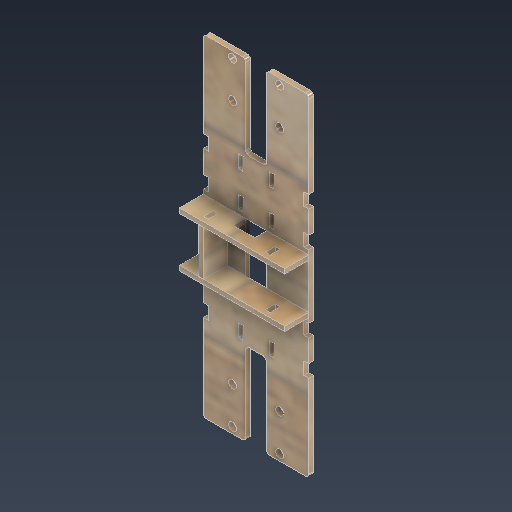
# Autodesk Inventor part: edited
Saved by Autodesk Inventor 2025.3 (Build 293356000, 356)
## iProperties
Created: 2025-09-03
Part Number: edited
Material: 木材 (楓木)
Document SubType Name: Modeling
Designer: 陳泓任
Density: 0.67 g/cm^3
Appearance: 天然楓木 - 深色亮面處理
Author: 陳泓任
Autodesk Inventor part; units mm, degrees
ref_plane "YZ Plane" through (0, 0, 0) normal (1, 0, 0) x (0, 1, 0)
ref_plane "XZ Plane" through (0, 0, 0) normal (0, 1, 0) x (-1, 0, 0)
ref_plane "XY Plane" through (0, 0, 0) normal (0, 0, 1) x (1, 0, 0)
sketch "草圖1" plane through (0, 0, 0) normal (0, 0, 1) x (1, 0, 0)
  line L0 (-33, -104) -> (33, 104) construction
  line L1 (33, -104) -> (-33, 104) construction
  line L2 (0, 128.5379) -> (0, -160.5456) construction
  circle A0 centre (-14.75, 100) radius 2.5
  circle A1 centre (14.75, 100) radius 2.5
  circle A2 centre (14.75, 77) radius 2.5
  circle A3 centre (-14.75, 77) radius 2.5
  line L3 (-33, 49.8787) -> (-30, 49.8787)
  line L4 (-30, 49.8787) -> (-30, 41.8787)
  line L5 (-30, 41.8787) -> (-33, 41.8787)
  line L6 (-33, 102) -> (-33, 49.8787)
  line L7 (-11.2, 49.8787) -> (-8.2, 49.8787)
  line L8 (-8.2, 49.8787) -> (-8.2, 41.8787)
  line L9 (-8.2, 41.8787) -> (-11.2, 41.8787)
  line L10 (-11.2, 41.8787) -> (-11.2, 49.8787)
  line L11 (33, 49.8787) -> (30, 49.8787)
  line L12 (30, 49.8787) -> (30, 41.8787)
  line L13 (30, 41.8787) -> (33, 41.8787)
  line L14 (11.2, 49.8787) -> (8.2, 49.8787)
  line L15 (8.2, 49.8787) -> (8.2, 41.8787)
  line L16 (8.2, 41.8787) -> (11.2, 41.8787)
  line L17 (11.2, 41.8787) -> (11.2, 49.8787)
  line L18 (33, 49.8787) -> (33, 102)
  line L19 (-33, 41.8787) -> (-33, 27.7533)
  line L20 (33, 27.7533) -> (33, 41.8787)
  line L21 (-4.5, 52) -> (4.5, 52)
  line L22 (6.5, 54) -> (6.5, 102)
  line L23 (-6.5, 102) -> (-6.5, 54)
  line L24 (-6.5, 52) -> (6.5, 104) construction
  line L25 (6.5, 52) -> (-6.5, 104) construction
  line L26 (31, 104) -> (8.5, 104)
  line L27 (-8.5, 104) -> (-31, 104)
  arc A4 (-6.5, 102) -> (-8.5, 104) centre (-8.5, 102) ccw
  arc A5 (8.5, 104) -> (6.5, 102) centre (8.5, 102) ccw
  arc A6 (-6.5, 54) -> (-4.5, 52) centre (-4.5, 54) ccw
  arc A7 (4.5, 52) -> (6.5, 54) centre (4.5, 54) ccw
  arc A8 (-31, 104) -> (-33, 102) centre (-31, 102) ccw
  arc A9 (33, 102) -> (31, 104) centre (31, 102) ccw
  line L28 (-82.8249, 0) -> (86.4934, 0) construction
  circle A10 centre (-14.75, -100) radius 2.5
  circle A11 centre (14.75, -100) radius 2.5
  circle A12 centre (14.75, -77) radius 2.5
  circle A13 centre (-14.75, -77) radius 2.5
  line L29 (-33, -49.8787) -> (-30, -49.8787)
  line L30 (-30, -49.8787) -> (-30, -41.8787)
  line L31 (-30, -41.8787) -> (-33, -41.8787)
  line L32 (-33, -102) -> (-33, -49.8787)
  line L33 (-11.2, -49.8787) -> (-8.2, -49.8787)
  line L34 (-8.2, -49.8787) -> (-8.2, -41.8787)
  line L35 (-8.2, -41.8787) -> (-11.2, -41.8787)
  line L36 (-11.2, -41.8787) -> (-11.2, -49.8787)
  line L37 (33, -49.8787) -> (30, -49.8787)
  line L38 (30, -49.8787) -> (30, -41.8787)
  line L39 (30, -41.8787) -> (33, -41.8787)
  line L40 (8.2, -41.8787) -> (11.2, -41.8787)
  line L41 (11.2, -41.8787) -> (11.2, -49.8787)
  line L42 (8.2, -49.8787) -> (8.2, -41.8787)
  line L43 (11.2, -49.8787) -> (8.2, -49.8787)
  line L44 (33, -49.8787) -> (33, -102)
  line L45 (8.2, -28.1) -> (8.2, -20.1)
  line L46 (8.2, -20.1) -> (11.2, -20.1)
  line L47 (11.2, -28.1) -> (8.2, -28.1)
  line L48 (11.2, -20.1) -> (11.2, -28.1)
  line L49 (30, -28.1) -> (30, -20.1)
  line L50 (30, -20.1) -> (33, -20.1)
  line L51 (33, -28.1) -> (30, -28.1)
  line L52 (-8.2, -28.1) -> (-8.2, -20.1)
  line L53 (-8.2, -20.1) -> (-11.2, -20.1)
  line L54 (-11.2, -28.1) -> (-8.2, -28.1)
  line L55 (-11.2, -20.1) -> (-11.2, -28.1)
  line L56 (-30, -28.1) -> (-30, -20.1)
  line L57 (-33, -28.1) -> (-30, -28.1)
  line L58 (-30, -20.1) -> (-33, -20.1)
  line L59 (-33, -41.8787) -> (-33, -28.1)
  line L60 (33, -28.1) -> (33, -41.8787)
  line L61 (-4.5, -52) -> (4.5, -52)
  line L62 (6.5, -54) -> (6.5, -102)
  line L63 (-6.5, -102) -> (-6.5, -54)
  line L64 (-6.5, -52) -> (6.5, -104) construction
  line L65 (6.5, -52) -> (-6.5, -104) construction
  line L66 (31, -104) -> (8.5, -104)
  line L67 (-8.5, -104) -> (-31, -104)
  arc A14 (-8.5, -104) -> (-6.5, -102) centre (-8.5, -102) ccw
  arc A15 (6.5, -102) -> (8.5, -104) centre (8.5, -102) ccw
  arc A16 (-4.5, -52) -> (-6.5, -54) centre (-4.5, -54) ccw
  arc A17 (6.5, -54) -> (4.5, -52) centre (4.5, -54) ccw
  arc A18 (-33, -102) -> (-31, -104) centre (-31, -102) ccw
  arc A19 (31, -104) -> (33, -102) centre (31, -102) ccw
  line L68 (-31, -104) -> (-8.5, -104)
  line L69 (8.5, -104) -> (31, -104)
  line L70 (-6.8, -17.1) -> (6.8, -17.1)
  line L71 (6.8, 17.1) -> (-6.8, 17.1)
  line L72 (-6.8, -17.1) -> (6.8, 17.1) construction
  line L73 (6.8, -17.1) -> (-6.8, 17.1) construction
  line L74 (12.065, 1.05) -> (12.065, 7.05)
  line L75 (-12.065, 7.05) -> (-12.065, 1.05)
  line L76 (-12.065, 1.05) -> (12.065, 7.05) construction
  line L77 (12.065, 1.05) -> (-12.065, 7.05) construction
  line L78 (-6.8, 17.1) -> (-6.8, 7.05)
  line L79 (-6.8, 1.05) -> (-6.8, -17.1)
  line L80 (6.8, -17.1) -> (6.8, 1.05)
  line L81 (6.8, 7.05) -> (6.8, 17.1)
  line L82 (12.065, 7.05) -> (6.8, 7.05)
  line L83 (6.8, 1.05) -> (12.065, 1.05)
  line L84 (-12.065, 1.05) -> (-6.8, 1.05)
  line L85 (-6.8, 7.05) -> (-12.065, 7.05)
  line L86 (-33, -28.1) -> (-33, -41.8787)
  line L87 (-33, -49.8787) -> (-33, -102)
  line L88 (33, -102) -> (33, -49.8787)
  line L89 (33, -41.8787) -> (33, -28.1)
  line L90 (-11.2, -41.8787) -> (-8.2, -49.8787) construction
  line L91 (-8.2, -41.8787) -> (-11.2, -49.8787) construction
  line L92 (-13.3213, -39.7574) -> (-6.0787, -39.7574) construction
  line L93 (-6.0787, -39.7574) -> (-6.0787, -52) construction
  line L94 (-6.0787, -52) -> (-13.3213, -52) construction
  line L95 (-13.3213, -52) -> (-13.3213, -39.7574) construction
  line L96 (-8.2, -41.8787) -> (-6.0787, -39.7574) construction
  circle A20 centre (-6.8, 17.1) radius 3 construction
  line L97 (-11.2, 27.7533) -> (-8.2, 27.7533)
  line L98 (-8.2, 27.7533) -> (-8.2, 19.7533)
  line L99 (-8.2, 19.7533) -> (-11.2, 19.7533)
  line L100 (-11.2, 19.7533) -> (-11.2, 27.7533)
  line L101 (-33, 27.7533) -> (-30, 27.7533)
  line L102 (-30, 27.7533) -> (-30, 19.7533)
  line L103 (-30, 19.7533) -> (-33, 19.7533)
  line L104 (11.2, 27.7533) -> (8.2, 27.7533)
  line L105 (8.2, 27.7533) -> (8.2, 19.7533)
  line L106 (8.2, 19.7533) -> (11.2, 19.7533)
  line L107 (11.2, 19.7533) -> (11.2, 27.7533)
  line L108 (33, 27.7533) -> (30, 27.7533)
  line L109 (30, 27.7533) -> (30, 19.7533)
  line L110 (30, 19.7533) -> (33, 19.7533)
  line L111 (-33, 19.7533) -> (-33, -20.1)
  line L112 (33, 19.7533) -> (33, -20.1)
  line L113 (-9.8, -17.1) -> (-14.1, -17.1) construction
  line L114 (-14.1, -17.1) -> (-14.1, -14.1) construction
  line L115 (-14.1, -14.1) -> (-9.8, -14.1) construction
  line L116 (-9.8, -14.1) -> (-9.8, -17.1) construction
  line L117 (-17.1, -20.1) -> (-6.8, -20.1) construction
  line L118 (-6.8, -20.1) -> (-6.8, -11.1) construction
  line L119 (-6.8, -11.1) -> (-17.1, -11.1) construction
  line L120 (-17.1, -11.1) -> (-17.1, -20.1) construction
  point P0 (0, 0)
  point P1 (0, 86.5078)
  point P2 (0, 78)
  point P3 (0, -86.5078)
  point P4 (0, -78)
  point P5 (0, 4.05)
  point P6 (12.065, 4.05)
  dimension "d56" = 6
  dimension "d0" = 66
  dimension "d1" = 208
  dimension "d6" = 5
  dimension "d8" = 29.5
  dimension "d9" = 23
  dimension "d10" = 3
  dimension "d11" = 8
  dimension "d13" = 3
  dimension "d14" = 18.8
  dimension "d22" = 13
  dimension "d23" = 4
  dimension "d24" = 2
  dimension "d25" = 2
  dimension "d26" = 34.2
  dimension "d27" = 13.6
  dimension "d28" = 6
  dimension "d30" = 24.13
  dimension "d31" = 10.05
  dimension "d53" = 3
  dimension "d54" = 52
  dimension "d57" = 3
  dimension "d58" = 3
  dimension "d71" = 4.3
  dimension "d72" = 3
  dimension "d73" = 3
  dimension "d74" = 3
  constraints: 242 end point, 60 symmetric about line, 42 parallel, 29 point on line, 24 point on circle, 22 perpendicular, 20 centre point, 16 collinear, 15 horizontal, 12 tangent, 11 equal length, 9 midpoint, 7 equal radius, 4 vertical, 1 coincident, 1 vertical alignment, 21 other
  measures "d0" distance of L0.end L1.end
  measures "d1" distance of L1.start L0.end
  measures "d6" diameter of A0
  measures "d8" distance of A2.centre A3.centre
  measures "d9" distance of A1.centre A2.centre
  measures "d10" distance of L4.end L5.end
  measures "d11" distance of L3.end L4.end
  measures "d13" distance of L7.start L7.end
  measures "d14" distance between parallel lines of L4 L10
  measures "d22" distance of L24.start L25.start
  measures "d23" distance from line of A0.centre L27
  measures "d24" radius of A4
  measures "d25" radius of A8
  measures "d26" distance of L70.end L71.start
  measures "d27" distance of L71.start L71.end
  measures "d28" distance of L74.start L74.end
  measures "d30" distance from line of point (12.065, 4.05) L75
  measures "d31" distance between parallel lines of L85 L71
  measures "d53" distance of L35.start L92.end
  measures "d54" distance between parallel lines of L27 L21
  measures "d57" distance of L97.start L97.end
  measures "d58" distance of L19.end L101.end
  measures "d71" distance of L114.end L115.end
  measures "d72" distance between parallel lines of L79 L116
  measures "d73" distance of L113.end L114.end
  measures "d74" distance between parallel lines of L113 L117
extrude "擠出1" add sketch "草圖1" along normal blind 3
sketch "草圖3" plane through (0, 0, 3) normal (0, 0, 1) x (1, 0, 0)
  line L0 (-88.1264, 0) -> (75.7938, 0)
  line L1 (0, 123.8394) -> (0, -129.4918)
  point P0 (0, 0)
  constraints: 4 end point, 2 point on line, 1 horizontal, 1 perpendicular
sketch "草圖5" plane through (0, 0, 3) normal (0, 0, 1) x (1, 0, 0)
  line L0 (-9.8, -17.1) -> (-13.8, -17.1)
  line L1 (-13.8, -17.1) -> (-13.8, -14.1)
  line L2 (-13.8, -14.1) -> (-9.8, -14.1)
  line L3 (-9.8, -14.1) -> (-9.8, -17.1)
  line L4 (6.8, -17.1) -> (-6.8, -17.1) projected
  line L5 (-6.8, -17.1) -> (-6.8, 1.05) projected
  line L6 (-9.8, 14.1) -> (-13.8, 14.1)
  line L7 (-13.8, 14.1) -> (-13.8, 17.1)
  line L8 (-13.8, 17.1) -> (-9.8, 17.1)
  line L9 (-9.8, 17.1) -> (-9.8, 14.1)
  line L10 (-6.8, 17.1) -> (6.8, 17.1) projected
  line L11 (-6.8, 7.05) -> (-6.8, 17.1) projected
  line L12 (0, 31.1544) -> (0, -25.4134)
  line L13 (9.8, -17.1) -> (13.8, -17.1)
  line L14 (13.8, -17.1) -> (13.8, -14.1)
  line L15 (13.8, -14.1) -> (9.8, -14.1)
  line L16 (9.8, -14.1) -> (9.8, -17.1)
  line L17 (13.8, 17.1) -> (9.8, 17.1)
  line L18 (13.8, 14.1) -> (13.8, 17.1)
  line L19 (9.8, 14.1) -> (13.8, 14.1)
  line L20 (9.8, 17.1) -> (9.8, 14.1)
  line L21 (-17.8, 2.175) -> (-20.8, 2.175)
  line L22 (-20.8, 2.175) -> (-20.8, 14.175)
  line L23 (-20.8, 14.175) -> (-17.8, 14.175)
  line L24 (-17.8, 14.175) -> (-17.8, 2.175)
  line L25 (17.8, 2.175) -> (20.8, 2.175)
  line L26 (20.8, 2.175) -> (20.8, 14.175)
  line L27 (20.8, 14.175) -> (17.8, 14.175)
  line L28 (17.8, 14.175) -> (17.8, 2.175)
  point P0 (0, 0)
  dimension "d60" = 4
  dimension "d61" = 3
  dimension "d62" = 3
  dimension "d64" = 3
  dimension "d65" = 3
  dimension "d66" = 3
  dimension "d67" = 12
  dimension "d68" = 11
  dimension "d101" = 0.075
  constraints: 50 end point, 12 symmetric about line, 6 parallel, 3 collinear, 3 horizontal, 3 perpendicular, 1 point on line, 1 vertical
  measures "d60" distance of L0.start L0.end
  measures "d61" distance between parallel lines of L3 L5
  measures "d62" distance of L0.end L1.end
  measures "d64" distance of L7.start L8.start
  measures "d65" distance between parallel lines of L9 L11
  measures "d66" distance of L22.end L23.end
  measures "d67" distance of L23.end L21.start
  measures "d68" distance between parallel lines of L5 L24
  measures "d101" distance between parallel lines of L23 L6
extrude "擠出4" cut sketch "草圖5" against normal up to next
sketch "草圖6" plane through (9.8, 17.1, 3) normal (0, -1, 0) x (1, 0, 0)
  line L0 (-16.6, 0) -> (-16.6, 7.5)
  line L1 (-16.6, 7.5) -> (-3, 7.5)
  line L2 (-16.6, -3) -> (-3, -3) projected
  line L3 (-3, 7.5) -> (-3, -3)
  line L4 (-16.6, -3) -> (-16.6, 0) projected
  line L5 (-19.6, 0) -> (-19.6, -3) projected
  line L6 (-19.6, -3) -> (-23.6, -3) projected
  line L7 (-23.6, 0) -> (-23.6, -3) projected
  line L8 (-23.6, 0) -> (-23.6, -3)
  line L9 (-19.6, -3) -> (-19.6, 0)
  line L10 (-19.6, 0) -> (-16.6, 0)
  line L11 (-19.6, -3) -> (-23.6, -3)
  line L12 (-23.6, 0) -> (-42.8, 0)
  line L13 (-42.8, 0) -> (-42.8, 15)
  line L14 (-14.3, 0) -> (-5.3, 0) projected
  line L15 (-42.8, 15) -> (-9.8, 15)
  line L16 (-9.8, 17.6895) -> (-9.8, 0) construction
  line L17 (-30.7, 12.1) -> (-27.7, 12.1)
  line L18 (-27.7, 12.1) -> (-27.7, 5.9)
  line L19 (-27.7, 5.9) -> (-30.7, 5.9)
  line L20 (-30.7, 5.9) -> (-30.7, 12.1)
  line L21 (0, 0) -> (0, -3)
  line L22 (0, -3) -> (4, -3)
  line L23 (4, 0) -> (4, -3)
  line L24 (4, 0) -> (4, -3)
  line L25 (0, -3) -> (0, 0)
  line L26 (0, 0) -> (-3, 0)
  line L27 (0, -3) -> (4, -3)
  line L28 (4, 0) -> (23.2, 0)
  line L29 (23.2, 15) -> (-9.8, 15)
  line L30 (11.1, 12.1) -> (8.1, 12.1)
  line L31 (8.1, 12.1) -> (8.1, 5.9)
  line L32 (8.1, 5.9) -> (11.1, 5.9)
  line L33 (11.1, 5.9) -> (11.1, 12.1)
  line L34 (23.2, 15) -> (23.2, 0)
  point P0 (-9.8, -3)
  point P1 (-9.8, -3)
  point P2 (-3, 0)
  dimension "d75" = 7.5
  dimension "d76" = 15
  dimension "d78" = 3
  dimension "d79" = 6.2
  dimension "d80" = 11.1
  dimension "d81" = 5.9
  dimension "d100" = 66
  constraints: 58 end point, 11 symmetric about line, 5 perpendicular, 4 parallel, 4 point on line, 3 horizontal, 2 midpoint, 2 vertical, 1 collinear
  measures "d75" distance between parallel lines of L14 L1
  measures "d76" distance of L12.end L13.end
  measures "d78" distance of L18.end L19.end
  measures "d79" distance of L17.end L18.end
  measures "d80" distance between parallel lines of L0 L18
  measures "d81" distance between parallel lines of L12 L19
  measures "d100" distance between parallel lines of L34 L13
extrude "擠出5" add sketch "草圖6" along normal blind 3 separate body contours L10 L5 L6 L7 L12 L13 L15 L29 L34 L28 L23 L22 L21 L26 L3 L1 L0
sketch "草圖8" plane through (9.8, -14.1, 3) normal (0, -1, 0) x (1, 0, 0)
  line L0 (-19.6, 0) -> (-19.6, -3) projected
  line L1 (-19.6, -3) -> (-23.6, -3) projected
  line L2 (-19.6, 0) -> (-19.6, -3)
  line L3 (-19.6, -3) -> (-23.6, -3)
  line L4 (-23.6, 0) -> (-23.6, -3) projected
  line L5 (-23.6, -3) -> (-23.6, 0)
  line L6 (-42.8, 15) -> (-42.8, 0) projected
  line L7 (-23.6, 0) -> (-42.8, 0)
  line L8 (23.2, 15) -> (-42.8, 15) projected
  line L9 (-42.8, 0) -> (-42.8, 15)
  line L10 (-42.8, 15) -> (23.2, 15)
  line L11 (23.2, 15) -> (23.2, 0)
  line L12 (23.2, 0) -> (4, 0)
  line L13 (4, 0) -> (4, -3)
  line L14 (4, -3) -> (0, -3) projected
  line L15 (4, -3) -> (0, -3)
  line L16 (0, -3) -> (0, 0)
  line L17 (-30.7, 12.1) -> (-27.7, 12.1) projected
  line L18 (-30.7, 12.1) -> (-27.7, 12.1)
  line L19 (-27.7, 12.1) -> (-27.7, 5.9)
  line L20 (-27.7, 5.9) -> (-30.7, 5.9)
  line L21 (-30.7, 5.9) -> (-30.7, 12.1)
  line L22 (8.1, 12.1) -> (11.1, 12.1) projected
  line L23 (8.1, 12.1) -> (11.1, 12.1)
  line L24 (11.1, 12.1) -> (11.1, 5.9)
  line L25 (11.1, 5.9) -> (8.1, 5.9)
  line L26 (8.1, 5.9) -> (8.1, 12.1)
  line L27 (11.1, 12.1) -> (11.1, 5.9) projected
  line L28 (-19.6, 0) -> (0, 0)
  line L29 (-16.6, 0) -> (-3, 0) projected
  point P0 (-9.8, -3)
  constraints: 40 end point, 7 perpendicular, 5 collinear, 4 parallel, 3 horizontal, 3 point on line, 1 vertical
extrude "擠出6" add sketch "草圖8" along normal blind 3 separate body
sketch "草圖7" plane through (-17.8, 2.175, 3) normal (-1, 0, 0) x (0, 0, 1)
  line L0 (-14.967, 10) -> (-14.967, 2)
  line L1 (0, 0) -> (-12.967, 0)
  line L2 (0, 12) -> (0, 12)
  line L3 (12, -19.35) -> (12, -16.35)
  line L4 (-8.967, 9) -> (-11.967, 9)
  line L5 (-11.967, 9) -> (-11.967, 3)
  line L6 (-11.967, 3) -> (-8.967, 3)
  line L7 (-8.967, 3) -> (-8.967, 9)
  line L8 (-14.967, 6) -> (-4.6244, 6) construction
  arc A0 (-12.967, 12) -> (-14.967, 10) centre (-12.967, 10) ccw
  arc A1 (-14.967, 2) -> (-12.967, 0) centre (-12.967, 2) ccw
  line L9 (0, -19.275) -> (15, -19.275) construction
  line L10 (6, -19.35) -> (6, -16.35)
  line L11 (12, 15) -> (12, 12)
  line L12 (-12.967, 12) -> (6, 12)
  line L13 (6, 12) -> (6, 15)
  line L14 (6, 15) -> (12, 15)
  line L15 (12, -19.35) -> (6, -19.35)
  line L16 (0, 12) -> (-3, 12) projected
  line L17 (12, 12) -> (15, 12)
  line L18 (15, 14.925) -> (15, 11.925) projected
  line L19 (15, 12) -> (15, -16.35)
  line L20 (15, -16.35) -> (12, -16.35)
  line L21 (6, -16.35) -> (0, -16.35)
  line L22 (0, -16.35) -> (0, 0)
  line L23 (0, -19.275) -> (0, -16.275) projected
  line L24 (15, -16.275) -> (15, -19.275) projected
  point P0 (-3, -2.175)
  dimension "d86" = 3
  dimension "d87" = 3
  dimension "d88" = 6
  dimension "d89" = 2
  dimension "d97" = 6
  dimension "d102" = 28.35
  dimension "d103" = 3
  dimension "d104" = 6
  dimension "d105" = 8.967
  dimension "d106" = 3
  constraints: 40 end point, 7 collinear, 6 perpendicular, 4 point on circle, 4 tangent, 3 vertical, 2 centre point, 2 horizontal, 2 parallel, 1 equal radius, 1 midpoint, 3 other
  measures "d86" distance between parallel lines of L0 L5
  measures "d87" distance of L5.end L6.end
  measures "d88" distance of L6.end L4.start
  measures "d89" radius of A0
  measures "d97" distance of L10.start L3.start
  measures "d102" distance of L17.end L19.end
  measures "d103" distance of L3.start L3.end
  measures "d104" distance of L10.end L21.end
  measures "d105" distance between parallel lines of L22 L7
  measures "d106" distance of L11.start L11.end
extrude "擠出7" add sketch "草圖7" along normal blind 3 separate body
